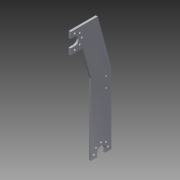
# Autodesk Inventor part: Leg_Link_Flame
Saved by Autodesk Inventor 2013 (Build 170138000, 138)
## iProperties
Created: 2014-04-20
Part Number: Leg_Link_Flame
Material: アルミニウム 6061
Document SubType Name: Modeling
Designer: andou
Density: 1 g/cm^3
Author: andou
Autodesk Inventor part; units mm, degrees
ref_plane "YZ Plane" through (0, 0, 0) normal (1, 0, 0) x (0, 1, 0)
ref_plane "XZ Plane" through (0, 0, 0) normal (0, 1, 0) x (-1, 0, 0)
ref_plane "XY Plane" through (0, 0, 0) normal (0, 0, 1) x (1, 0, 0)
sketch "スケッチ1" plane through (0, 0, 0) normal (1, 0, 0) x (0, 1, 0)
  line L0 (-20, 60) -> (20, 60)
  line L1 (20, 60) -> (20, -60)
  line L2 (20, -60) -> (-20, -60)
  line L3 (-20, -60) -> (-20, 60)
  point P0 (0, 0)
  dimension "d0" = 40
  dimension "d2" = 20
  dimension "d3" = 120
  dimension "d4" = 60
  constraints: 8 end point, 2 parallel, 1 horizontal, 1 perpendicular
  measures "d0" distance between parallel lines of L1 L3
  measures "d2" distance from line of L1 point (0, 0)
  measures "d3" distance between parallel lines of L2 L0
  measures "d4" distance from line of L2 point (0, 0)
extrude "押し出し1" add sketch "スケッチ1" along normal blind 2
sketch "スケッチ2" plane through (2, 0, 0) normal (1, 0, 0) x (0, 0, -1)
  line L0 (-60, 20) -> (-60, -20) projected
  line L1 (-60, -20) -> (60, -20) projected
  line L2 (60, -20) -> (60, 20) projected
  line L3 (60, 20) -> (-60, 20) projected
  line L4 (-60, 6.6025) -> (-10, 20)
  line L5 (-40, -20) -> (-40, -8.0385)
  line L6 (-40, -8.0385) -> (-10, 0)
  line L7 (-10, 0) -> (60, 0)
  point P0 (0, 0)
  dimension "d7" = 20
  dimension "d8" = 20
  dimension "d9" = 70
  dimension "d10" = 15
  dimension "d11" = 70
  constraints: 8 end point, 3 point on line, 2 perpendicular, 1 midpoint, 1 parallel
  measures "d7" distance between parallel lines of L3 L7
  measures "d8" distance between parallel lines of L0 L5
  measures "d9" distance of L6.end L7.end
  measures "d10" angle of L7 L6
  measures "d11" distance from line of L2 L4.end
extrude "押し出し2" cut sketch "スケッチ2" against normal blind 2 contours L4 L3 L2 L7 L6 L5 L1 L0 keep common part
sketch "スケッチ3" plane through (2, 0, 0) normal (1, 0, 0) x (0, 0, -1)
  line L0 (60, 0) -> (-10, 0) projected
  line L1 (60, 0) -> (60, 20) projected
  line L2 (-60, 6.6025) -> (-60, -20) projected
  line L3 (-60, -20) -> (-40, -20) projected
  line L4 (-54, -20) -> (-46, -20)
  line L5 (-46, -20) -> (-46, -16)
  line L6 (-54, -16) -> (-54, -20)
  line L7 (60, 14) -> (56, 14)
  line L8 (56, 6) -> (60, 6)
  line L9 (60, 6) -> (60, 14)
  arc A0 (-46, -16) -> (-54, -16) centre (-50, -16) ccw
  arc A1 (56, 14) -> (56, 6) centre (56, 10) ccw
  point P0 (0, 0)
  dimension "d14" = 8
  dimension "d16" = 8
  dimension "d19" = 4
  dimension "d20" = 4
  dimension "d21" = 10
  dimension "d22" = 4
  dimension "d23" = 4
  dimension "d24" = 10
  dimension "d26" = 4
  dimension "d27" = 4
  constraints: 12 end point, 4 point on circle, 2 centre point, 2 horizontal, 2 parallel, 2 point on line, 1 perpendicular
  measures "d14" distance between parallel lines of L5 L6
  measures "d16" distance between parallel lines of L7 L8
  measures "d19" radius of A1
  measures "d20" radius of A0
  measures "d21" distance from line of L2 A0.centre
  measures "d22" distance from line of A0.centre L4
  measures "d23" distance of L6.start L4.start
  measures "d24" distance from line of L0 A1.centre
  measures "d26" distance of L7.start L7.end
  measures "d27" distance from line of L1 A1.centre
extrude "押し出し3" cut sketch "スケッチ3" against normal blind 2
sketch "スケッチ4" plane through (2, 0, 0) normal (1, 0, 0) x (0, 0, -1)
  arc A0 (-46, -16) -> (-54, -16) centre (-50, -16) ccw projected
  arc A1 (56, 14) -> (56, 6) centre (56, 10) ccw projected
  circle A2 centre (-43, -16) radius 1
  circle A3 centre (56, 17) radius 1
  point P0 (0, 0)
  dimension "d30" = 2
  dimension "d32" = 7
  dimension "d33" = 0
  dimension "d34" = 7
  dimension "d35" = 0
  constraints: 2 centre point, 1 equal radius
  measures "d30" diameter of A3
  measures "d32" distance of A1.centre A3.centre
  measures "d33" horizontal distance of A1.centre A3.centre
  measures "d34" distance of A0.centre A2.centre
  measures "d35" vertical distance of A0.centre A2.centre
hole "穴1" at (2, 17, -56) at (2, -16, 43) direction (-1, 0, 0) diameter 2 end through all
pattern_circular "円形状パターン1" count 5 over 180 about axis through (2, 10, -56) along (1, 0, 0) of "穴1"
pattern_circular "円形状パターン2" count 5 over 180 about axis through (2, -16, 50) along (1, 0, 0) of "穴1"
sketch "スケッチ5" plane through (2, 0, 0) normal (1, 0, 0) x (0, 0, -1)
  line L0 (60, 14) -> (60, 20) projected
  line L1 (60, 20) -> (-10, 20) projected
  circle A0 centre (-5, 15) radius 1
  circle A1 centre (5, 15) radius 1
  point P0 (0, 0)
  dimension "d49" = 10
  dimension "d51" = 5
  dimension "d52" = 5
  dimension "d53" = 2
  dimension "d54" = 55
  constraints: 2 centre point, 1 equal radius
  measures "d49" distance of A1.centre A0.centre
  measures "d51" distance from line of L1 A0.centre
  measures "d52" distance from line of L1 A1.centre
  measures "d53" diameter of A1
  measures "d54" distance from line of L0 A1.centre
hole "穴2" at (2, 15, -5) at (2, 15, 5) direction (-1, 0, 0) diameter 1.5 end through all
